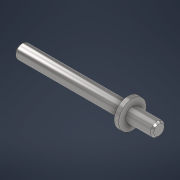
# Autodesk Inventor part: 18102021-002-05
Saved by Autodesk Inventor 2021 (Build 250183000, 183)
## iProperties
Created: 2021-10-15
Part Number: 18102021-002-05
Material: Stainless Steel
Document SubType Name: Modeling
Designer: DuctopwH
Density: 8 g/cm^3
Appearance: Semi-Polished
Author: DuctopwH
Autodesk Inventor part; units mm, degrees
ref_plane "YZ Plane" through (0, 0, 0) normal (1, 0, 0) x (0, 1, 0)
ref_plane "XZ Plane" through (0, 0, 0) normal (0, 1, 0) x (-1, 0, 0)
ref_plane "XY Plane" through (0, 0, 0) normal (0, 0, 1) x (1, 0, 0)
sketch "Sketch1" plane through (0, 0, 0) normal (0, 0, 1) x (1, 0, 0)
  line L0 (0, 0) -> (-40, 0)
  line L1 (-40, 0) -> (-40, 1.5)
  line L2 (-40, 1.5) -> (-39.5, 2)
  line L3 (-39.5, 2) -> (-9, 2)
  line L4 (-9, 2) -> (-9, 4)
  line L5 (-9, 4) -> (-7.7, 4)
  line L6 (-7.7, 4) -> (-7.7, 2)
  line L7 (-7.7, 2) -> (-0.5, 2)
  line L8 (-0.5, 2) -> (0, 1.5)
  line L9 (0, 1.5) -> (0, 0)
  dimension "d0" = 4
  dimension "d1" = 8
  dimension "d2" = 40
  dimension "d3" = 0.5
  dimension "d4" = 45
  dimension "d5" = 45
  dimension "d6" = 0.5
  dimension "d7" = 1.3
  dimension "d8" = 7.7
  constraints: 20 end point, 4 perpendicular, 2 parallel, 2 point on line, 1 horizontal
  measures "d0" diameter of L3 L0
  measures "d1" diameter of L5 L0
  measures "d2" distance between parallel lines of L9 L1
  measures "d3" horizontal distance of L2.end L1.end
  measures "d4" angle of L1 L2
  measures "d5" angle of L7 L8
  measures "d6" horizontal distance of L8.end L7.end
  measures "d7" distance between parallel lines of L6 L4
  measures "d8" distance between parallel lines of L9 L6
revolve "Revolution1" add sketch "Sketch1" angle 360 about axis through (0, 0, 0) along (-1, 0, 0)
body "Solid1"
